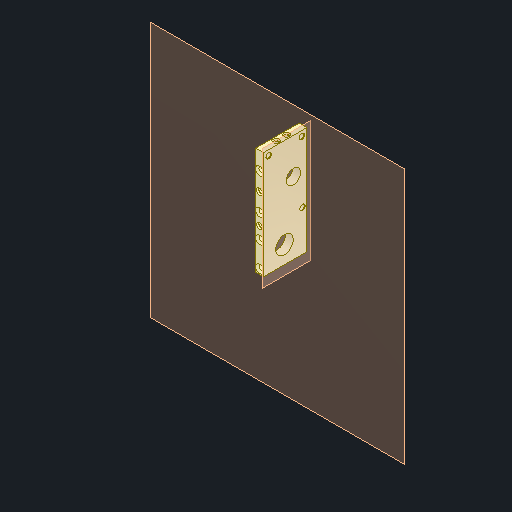
# Autodesk Inventor part: left_gear_holder
Saved by Autodesk Inventor 2023 (Build 270158000, 158)
## iProperties
Created: 2024-04-23
Part Number: left_gear_holder
Material: Nylon 6/6
Document SubType Name: Modeling
Designer: szymo
Density: 1.13 g/cm^3
Appearance: Nylon 6
Mass: 14.9327 g
Surface Area: 88.4291 cm^2
Volume: 13.2148 cm^3
Author: szymo
Autodesk Inventor part; units mm, degrees
ref_plane "YZ Plane" through (0, 0, 0) normal (1, 0, 0) x (0, 1, 0)
ref_plane "XZ Plane" through (0, 0, 0) normal (0, 1, 0) x (-1, 0, 0)
ref_plane "Work Plane1" through (0, 0, 0) normal (0, 0, 1) x (1, 0, 0)
sketch "Sketch1" plane through (0, 0, 0) normal (0, 0, 1) x (1, 0, 0)
  line L0 (23.5, 88.5) -> (-23.5, 88.5) projected
  line L1 (-23.5, 88.5) -> (-23.5, 36.5) projected
  line L2 (-26.5, 33.5) -> (-89, 33.5) projected
  line L3 (-89, 33.5) -> (-89, -72.5) projected
  line L4 (-89, -72.5) -> (-77, -72.5) projected
  line L5 (-74, -75.5) -> (-74, -93.5) projected
  line L6 (-74, -93.5) -> (74, -93.5) projected
  line L7 (74, -93.5) -> (74, -75.5) projected
  line L8 (77, -72.5) -> (89, -72.5) projected
  line L9 (89, -72.5) -> (89, 33.5) projected
  line L10 (89, 33.5) -> (26.5, 33.5) projected
  line L11 (23.5, 36.5) -> (23.5, 88.5) projected
  line L12 (-4.5, 81.5) -> (-4.5, 36.5) projected
  line L13 (-7.5, 33.5) -> (-13.5, 33.5) projected
  line L14 (-16.5, 36.5) -> (-16.5, 81.5) projected
  line L15 (7.5, 84.5) -> (13.5, 84.5) projected
  line L16 (16.5, 81.5) -> (16.5, 36.5) projected
  line L17 (13.5, 33.5) -> (7.5, 33.5) projected
  line L18 (4.5, 36.5) -> (4.5, 81.5) projected
  line L19 (-13.5, 84.5) -> (-7.5, 84.5) projected
  line L20 (16.5, 88.5) -> (22.5, 88.5)
  line L21 (22.5, 88.5) -> (22.5, 3.75)
  line L22 (22.5, 3.75) -> (16.5, 3.75)
  line L23 (16.5, 3.75) -> (16.5, 88.5)
  line L24 (59.9, 4.75) -> (32.2, 4.75)
  arc A0 (13.5, 33.5) -> (16.5, 36.5) centre (13.5, 36.5) ccw projected
  arc A1 (4.5, 36.5) -> (7.5, 33.5) centre (7.5, 36.5) ccw projected
  arc A2 (7.5, 84.5) -> (4.5, 81.5) centre (7.5, 81.5) ccw projected
  arc A3 (16.5, 81.5) -> (13.5, 84.5) centre (13.5, 81.5) ccw projected
  arc A4 (-4.5, 81.5) -> (-7.5, 84.5) centre (-7.5, 81.5) ccw projected
  arc A5 (-7.5, 33.5) -> (-4.5, 36.5) centre (-7.5, 36.5) ccw projected
  arc A6 (-16.5, 36.5) -> (-13.5, 33.5) centre (-13.5, 36.5) ccw projected
  arc A7 (-13.5, 84.5) -> (-16.5, 81.5) centre (-13.5, 81.5) ccw projected
  arc A8 (-26.5, 33.5) -> (-23.5, 36.5) centre (-26.5, 36.5) ccw projected
  arc A9 (-74, -75.5) -> (-77, -72.5) centre (-77, -75.5) ccw projected
  arc A10 (77, -72.5) -> (74, -75.5) centre (77, -75.5) ccw projected
  arc A11 (23.5, 36.5) -> (26.5, 33.5) centre (26.5, 36.5) ccw projected
  circle A12 centre (39.125, 25.9125) radius 1.0065 projected
  circle A13 centre (72.95, 12.275) radius 1.0065 projected
  circle A14 centre (-39.125, 12.3375) radius 1.0065 projected
  circle A15 centre (-72.95, 25.975) radius 1.0065 projected
  circle A16 centre (-72.95, 12.275) radius 1.0065 projected
  circle A17 centre (-39.125, 25.9125) radius 1.0065 projected
  circle A18 centre (72.95, 25.975) radius 1.0065 projected
  circle A19 centre (39.125, 12.3375) radius 1.0065 projected
  circle A20 centre (-42.4984, -44.6666) radius 1.2295 projected
  circle A21 centre (-79, -42.3889) radius 1.2295 projected
  circle A22 centre (-19.5, 28.875) radius 1.2295 projected
  circle A23 centre (19.5, 9.55) radius 1.2295 projected
  circle A24 centre (19.5, 47.3) radius 1.2295 projected
  circle A25 centre (-19.5, 47.3) radius 1.2295 projected
  circle A26 centre (0, 74.7) radius 1.2295 projected
  circle A27 centre (-19.4231, 74.8077) radius 1.2295 projected
  circle A28 centre (19.5, 74.7) radius 1.2295 projected
  circle A29 centre (0, 49.05) radius 1.2295 projected
  circle A30 centre (19.5, 28.875) radius 1.2295 projected
  circle A31 centre (0, 19.125) radius 1.2295 projected
  circle A32 centre (-19.5, 9.55) radius 1.2295 projected
  circle A33 centre (42.5, -44.6649) radius 1.2295 projected
  circle A34 centre (79, -42.3889) radius 1.2295 projected
  circle A35 centre (21.5, -85.5) radius 1.8 projected
  circle A36 centre (-64.5, -85.5) radius 1.8 projected
  circle A37 centre (-21.5, -85.5) radius 1.8 projected
  circle A38 centre (64.5, -85.5) radius 1.8 projected
  line L25 (-57, -78.5) -> (-82, -60.2553) projected
  line L26 (-82, -60.2553) -> (-82, -45.3889) projected
  line L27 (-76, -45.3889) -> (-45.4984, -47.6666) projected
  line L28 (-21.1, -27.9) -> (-21.1, -21.9) projected
  line L29 (-45.4984, -41.6666) -> (-76, -39.3889) projected
  line L30 (-82, -39.3889) -> (-82, 4.75) projected
  line L31 (30.3333, 4.75) -> (82, 4.75) projected
  line L32 (82, 4.75) -> (82, -39.3889) projected
  line L33 (76, -39.3889) -> (45.5, -41.6649) projected
  line L34 (21.1, -21.9) -> (21.1, -27.9) projected
  line L35 (45.5, -47.6649) -> (76, -45.3889) projected
  line L36 (82, -45.3889) -> (82, -60.2553) projected
  line L37 (82, -60.2553) -> (57, -78.5) projected
  line L38 (57, -78.5) -> (57, -87.5) projected
  arc A39 (55, -89.5) -> (57, -87.5) centre (55, -87.5) ccw projected
  line L39 (55, -89.5) -> (31, -89.5) projected
  arc A40 (29, -87.5) -> (31, -89.5) centre (31, -87.5) ccw projected
  line L40 (29, -87.5) -> (29, -78.5) projected
  line L41 (14, -78.5) -> (14, -87.5) projected
  arc A41 (12, -89.5) -> (14, -87.5) centre (12, -87.5) ccw projected
  line L42 (12, -89.5) -> (-12, -89.5) projected
  arc A42 (-14, -87.5) -> (-12, -89.5) centre (-12, -87.5) ccw projected
  line L43 (-14, -87.5) -> (-14, -78.5) projected
  line L44 (-29, -78.5) -> (-29, -87.5) projected
  arc A43 (-31, -89.5) -> (-29, -87.5) centre (-31, -87.5) ccw projected
  line L45 (-31, -89.5) -> (-55, -89.5) projected
  arc A44 (-57, -87.5) -> (-55, -89.5) centre (-55, -87.5) ccw projected
  line L46 (-57, -87.5) -> (-57, -78.5) projected
  line L47 (-69.95, 28.9125) -> (-42.125, 28.9125) projected
  line L48 (-42.125, 28.9125) -> (-42.125, 9.275) projected
  line L49 (-42.125, 9.275) -> (-69.95, 9.275) projected
  line L50 (-69.95, 9.275) -> (-69.95, 28.9125) projected
  line L51 (-16.5, 9.75) -> (-16.5, 28.5) projected
  line L52 (-16.5, 28.5) -> (-4.5, 28.5) projected
  line L53 (-4.5, 28.5) -> (-4.5, 9.75) projected
  line L54 (-4.5, 9.75) -> (-16.5, 9.75) projected
  line L55 (69.95, 9.3375) -> (42.125, 9.3375) projected
  line L56 (42.125, 9.3375) -> (42.125, 28.975) projected
  line L57 (42.125, 28.975) -> (69.95, 28.975) projected
  line L58 (69.95, 28.975) -> (69.95, 9.3375) projected
  line L59 (4.5, 9.75) -> (4.5, 28.5) projected
  line L60 (4.5, 28.5) -> (16.5, 28.5) projected
  line L61 (16.5, 28.5) -> (16.5, 9.75) projected
  line L62 (16.5, 9.75) -> (4.5, 9.75) projected
  line L63 (45.5, -41.6649) -> (27.1, -21.9) projected
  line L64 (27.1, -21.9) -> (30.3333, 4.75) projected
  line L65 (-45.4984, -47.6666) -> (-29, -78.5) projected
  line L66 (-82, 4.75) -> (-30.3333, 4.75) projected
  line L67 (-30.3333, 4.75) -> (-27.1, -21.9) projected
  line L68 (-27.1, -21.9) -> (-45.4984, -41.6666) projected
  line L69 (29, -78.5) -> (45.5, -47.6649) projected
  line L70 (-14, -78.5) -> (-39, -45.3279) projected
  line L71 (-39, -44.2124) -> (-21.1, -27.9) projected
  line L72 (-21.1, -21.9) -> (-24.3333, 4.75) projected
  line L73 (-24.3333, 4.75) -> (24.3333, 4.75) projected
  line L74 (24.3333, 4.75) -> (21.1, -21.9) projected
  line L75 (21.1, -27.9) -> (39.5, -44.6649) projected
  line L76 (39.5, -44.6649) -> (14, -78.5) projected
  circle A45 centre (-78, -67.1725) radius 1.2295 projected
  circle A46 centre (78, -67.1725) radius 1.2295 projected
  line L77 (-22.5, 28.9125) -> (-22.5, 9.55) projected
  line L78 (-22.5, 9.55) -> (-36.125, 9.55) projected
  line L79 (-36.125, 9.55) -> (-36.125, 28.9125) projected
  line L80 (-36.125, 28.9125) -> (-22.5, 28.9125) projected
  line L81 (76, -45.3889) -> (82, -45.3889) projected
  line L82 (82, -39.3889) -> (76, -39.3889) projected
  line L83 (36.125, 9.275) -> (22.5, 9.275) projected
  line L84 (22.5, 9.275) -> (22.5, 28.9125) projected
  line L85 (22.5, 28.9125) -> (36.125, 28.9125) projected
  line L86 (36.125, 28.9125) -> (36.125, 9.275) projected
  line L87 (-86, 28.975) -> (-75.95, 28.975) projected
  line L88 (-75.95, 28.975) -> (-75.95, 9.275) projected
  line L89 (-75.95, 9.275) -> (-86, 9.275) projected
  line L90 (-86, 9.275) -> (-86, 28.975) projected
  line L91 (-82, -45.3889) -> (-76, -45.3889) projected
  line L92 (-76, -39.3889) -> (-82, -39.3889) projected
  line L93 (75.95, 28.975) -> (86, 28.975) projected
  line L94 (86, 28.975) -> (86, 9.275) projected
  line L95 (86, 9.275) -> (75.95, 9.275) projected
  line L96 (75.95, 9.275) -> (75.95, 28.975) projected
  line L97 (-39, -45.3279) -> (-39, -44.2124) projected
  circle A47 centre (-24.1, -73.1) radius 1.2295 projected
  circle A48 centre (24.1, -24.9) radius 1.2295 projected
  circle A49 centre (-24.1, -24.9) radius 1.2295 projected
  circle A50 centre (24.1, -73.1) radius 1.2295 projected
  point P0 (0, 0)
  point P1 (7.5, 81.5)
  point P2 (13.5, 81.5)
  point P3 (-7.5, 81.5)
  point P4 (-13.5, 81.5)
  point P5 (-77, -75.5)
  point P6 (39, -44.2094)
  point P7 (-79, -67.8878)
  point P8 (-79, -66.4572)
  point P9 (22.5, 12.275)
  point P10 (22.5, 25.9125)
  point P11 (7.5, 81.5)
  point P12 (13.5, 81.5)
  point P13 (-7.5, 81.5)
  point P14 (-13.5, 81.5)
  dimension "d0" = 1
  dimension "d1" = 1
  constraints: 10 end point, 2 horizontal, 2 parallel, 1 collinear, 1 perpendicular, 1 point on line, 2 other
  measures "d0" distance between parallel lines of L21 L11
  measures "d1" distance between parallel lines of L24 L22
ref_plane "Work Plane2" through (-89, -40.3889, 33.5) normal (0, 0, 1) x (1, 0, 0)
extrude "Extrusion1" add sketch "Sketch1" along normal up to surface (33.5 mm away) contours L21 L73 L23 L16 L0 | L21 L22 L23 L73 | A23 | A24 | A28 | A30
sketch "Sketch2" plane through (22.5, 3.75, 0) normal (1, 0, 0) x (0, 0, -1)
  circle A0 centre (-17.375, 15.375) radius 6.75 projected
  circle A1 centre (-10.5, 57.25) radius 5.5 projected
  point P0 (0, -3.75)
  dimension "d8" = 11
  measures "d8" diameter of A1
extrude "Extrusion2" cut sketch "Sketch2" against normal up to next
sketch "Sketch3" plane through (16.5, 3.75, 0) normal (-1, 0, 0) x (0, 0, 1)
  circle A0 centre (23.4363, 30.1825) radius 2 projected
  point P0 (0, -3.75)
extrude "Extrusion3" cut sketch "Sketch3" against normal blind 5
ref_plane "Work Plane3" through (23.5, 3.75, 0) normal (1, 0, 0) x (0, 0, -1)
sketch "Sketch4" plane through (23.5, 3.75, 0) normal (1, 0, 0) x (0, 0, -1)
  circle A0 centre (-29.5, 80.75) radius 1.8 projected
  circle A1 centre (-3.5, 33.25) radius 1.8 projected
  circle A2 centre (-4, 80.75) radius 1.8 projected
  point P0 (0, -3.75)
hole "Hole1" at (23.5, 37, 3.5) at (23.5, 84.5, 4) at (23.5, 84.5, 29.5) direction (-1, 0, 0) diameter 3.6 end through all countersink diameter 6.2 countersink angle 90 clearance for "Countersunk Flat Head Screw ISO 2009/7046" size "M3" standard "ISO"
sketch "Sketch5" plane through (16.5, 3.75, 33.5) normal (0, 0, 1) x (1, 0, 0)
  circle A0 centre (-36, 5.8) radius 1.8 projected
  circle A1 centre (-36, 25.125) radius 1.8 projected
  circle A2 centre (-36, 43.55) radius 1.8 projected
  circle A3 centre (-35.9231, 71.0577) radius 1.8 projected
  circle A4 centre (-16.5, 45.3) radius 3.3 projected
  circle A5 centre (-16.5, 15.375) radius 3.3 projected
  circle A6 centre (-16.5, 70.95) radius 3.3 projected
  line L0 (-12, 2) -> (-21, 2) projected
  line L1 (-12, 84.75) -> (-12, 2) projected
  line L2 (-21, 84.75) -> (-12, 84.75) projected
  line L3 (-21, 2) -> (-21, 84.75) projected
  line L4 (-16.5, 2) -> (-16.5, 84.75)
  circle A7 centre (3, 5.8) radius 1.8
  circle A8 centre (3, 25.125) radius 1.8
  circle A9 centre (3, 43.55) radius 1.8
  circle A10 centre (2.9231, 71.0577) radius 1.8
  circle A11 centre (-16.5, 30.7161) radius 2.3 projected
  circle A12 centre (-16.5, 59.25) radius 2.3 projected
  point P0 (-16.5, -3.75)
  constraints: 4 centre point, 4 coincident, 4 symmetric about line, 2 end point, 2 midpoint, 4 other
hole "Hole2" at (19.5, 9.55, 33.5) at (19.5, 28.875, 33.5) at (19.5, 47.3, 33.5) at (19.4231, 74.8077, 33.5) direction (0, 0, -1) diameter 3.6 end through all countersink diameter 6.3 countersink angle 90 clearance for "Countersunk Flat Head Screw ISO 2009/7046" size "M3" standard "ISO"
sketch "Sketch7" plane through (16.5, 88.5, 0) normal (0, 1, 0) x (1, 0, 0)
  line L0 (0, -33.5) -> (6, -33.5) projected
  line L1 (6, 0) -> (6, -33.5) projected
  line L2 (6, 0) -> (0, 0) projected
  line L3 (0, 0) -> (0, -33.5) projected
  circle A0 centre (-16.5, -12.675) radius 2 projected
  circle A1 centre (-16.5, -20.825) radius 2 projected
  line L4 (-16.5, -20.825) -> (6, -20.825)
  line L5 (-16.5, -12.675) -> (6, -12.675)
  line L6 (6, -5) -> (6, -16) projected
  point P0 (-16.5, 0)
  point P1 (3, -20.825)
  point P2 (3, -12.675)
  constraints: 4 end point, 4 point on line, 2 perpendicular
hole "Hole4" at (19.5, 88.5, 20.825) at (19.5, 88.5, 12.675) direction (0, -1, 0) diameter 4 depth 6 counterbore diameter 4.6 counterbore depth 1.5
sketch "Sketch8" plane through (19.5, 47.3, 33.5) normal (0, 0, 1) x (1, 0, 0)
  circle A0 centre (-39, -9.2125) radius 2.3 projected
  circle A1 centre (-39, 13.7) radius 2.3 projected
  arc A2 (3, 0.9605) -> (-3, 0.9605) centre (0, 0) ccw projected
  line L0 (3, 26.8331) -> (3, 0.9605) projected
  arc A3 (-3, 26.3338) -> (3, 26.8331) centre (-0.0769, 27.5077) ccw projected
  line L1 (-3, 0.9605) -> (-3, 26.3338) projected
  arc A4 (-3, -0.9605) -> (3, -0.9605) centre (0, 0) ccw projected
  line L2 (-3, -17.4645) -> (-3, -0.9605) projected
  arc A5 (3, -17.4645) -> (-3, -17.4645) centre (0, -18.425) ccw projected
  line L3 (3, -0.9605) -> (3, -17.4645) projected
  line L4 (-39, 13.7) -> (3, 13.7)
  line L5 (3, 19.2) -> (3, 8.2) projected
  line L6 (-39, -9.2125) -> (3, -9.2125)
  circle A6 centre (0, -18.425) radius 1.8 projected
  line L7 (0, -18.425) -> (-0.0769, 27.5077)
  point P0 (-19.5, -47.3)
  point P1 (-0.0538, 13.7)
  point P2 (-0.0154, -9.2125)
  constraints: 6 end point, 4 point on line, 2 midpoint
hole "Hole5" at (19.4462, 61, 33.5) at (19.4846, 38.0875, 33.5) direction (0, 0, -1) diameter 4 depth 6 counterbore diameter 4.6 counterbore depth 1.5
sketch "Sketch9" plane through (16.5, 3.75, 0) normal (0, -1, 0) x (1, 0, 0)
  line L0 (0, 0) -> (0, 33.5) projected
  line L1 (0, 0) -> (6, 0) projected
  line L2 (6, 0) -> (6, 33.5) projected
  line L3 (6, 33.5) -> (0, 33.5) projected
  point P0 (-16.5, 0)
extrude "Extrusion4" cut sketch "Sketch9" against normal blind 2
body "Solid1"
